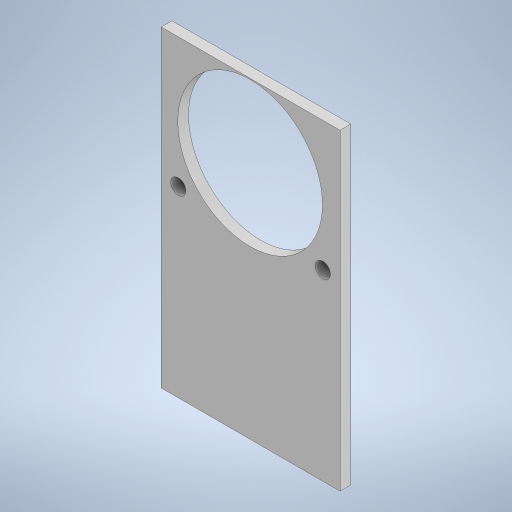
# Autodesk Inventor part: Motor_Cover
Saved by Autodesk Inventor 2023.5 (Build 275446020, 446B)
## iProperties
Created: 2025-04-14
Part Number: Motor_Cover
Material: Generic
Document SubType Name: Modeling
Designer: Lucky Sah
Density: 1 g/cm^3
Appearance: Default
Author: Lucky Sah
Autodesk Inventor part; units mm, degrees
ref_plane "YZ Plane" through (0, 0, 0) normal (1, 0, 0) x (0, 1, 0)
ref_plane "XZ Plane" through (0, 0, 0) normal (0, 1, 0) x (-1, 0, 0)
ref_plane "XY Plane" through (0, 0, 0) normal (0, 0, 1) x (1, 0, 0)
sketch "Sketch1" plane through (0, 0, 0) normal (0, 0, 1) x (1, 0, 0)
  line L0 (-58.7621, -16.5299) -> (-25.3621, -16.5299)
  line L1 (-25.3621, -16.5299) -> (-25.3621, 41.8701)
  line L2 (-25.3621, 41.8701) -> (-58.7621, 41.8701)
  line L3 (-58.7621, 41.8701) -> (-58.7621, -16.5299)
  circle A0 centre (-42.1621, 28.1701) radius 13.5
  circle A1 centre (-55.5621, 17.6701) radius 1.4
  circle A2 centre (-28.5621, 17.6701) radius 1.4
  point P0 (0, 0)
  dimension "d1" = 33.4
  dimension "d17" = 27
  dimension "d18" = 13.7
  dimension "d21" = 3.2
  dimension "d22" = 2.8
  dimension "d27" = 58.4
  dimension "d28" = 10.5
  dimension "d29" = 10.5
  dimension "d30" = 2.8
  dimension "d31" = 27
  constraints: 8 end point, 3 centre point, 2 parallel, 1 horizontal, 1 perpendicular
  measures "d1" distance between parallel lines of L1 L3
  measures "d17" diameter of A0
  measures "d18" distance from line of A0.centre L2
  measures "d21" distance from line of L3 A1.centre
  measures "d22" diameter of A2
  measures "d27" distance between parallel lines of L0 L2
  measures "d28" vertical distance of A2.centre A0.centre
  measures "d29" vertical distance of A1.centre A0.centre
  measures "d30" diameter of A1
  measures "d31" distance of A2.centre A1.centre
extrude "Extrusion1" add sketch "Sketch1" along normal blind 2
body "Solid1"
